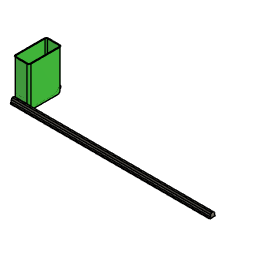
main v3 (Autodesk Fusion 360 archive; units mm, degrees)
design "main"
part number: Configuration 1
Autodesk Fusion 360 part; units mm, degrees
sketch "Sketch1" plane through (0, 0, 0) normal (0, 0, 1) x (1, 0, 0)
  line L0 (0, 0) -> (24, 0)
  line L1 (24, 0) -> (24, 50)
  line L2 (24, 50) -> (0, 50)
  line L3 (0, 50) -> (0, 0)
  line L4 (0.25, 49.75) -> (23.75, 49.75)
  line L5 (23.75, 49.75) -> (23.75, 0.25)
  line L6 (23.75, 0.25) -> (0.25, 0.25)
  line L7 (0.25, 0.25) -> (0.25, 49.75)
  dimension "d5" = 24
  dimension "d6" = 50
  dimension "d8" = 0.25
  dimension "d9" = 0.25
  dimension "d10" = 0.25
  dimension "d11" = 0.25
  constraint horizontal L0
  constraint vertical L1
  constraint horizontal L2
  constraint vertical L3
  constraint coincident L0.start L3.end
  constraint horizontal L4
  constraint vertical L5
  constraint horizontal L6
  constraint vertical L7
  measures "d5" distance of L0.start L0.end
  measures "d6" distance of L0.start L2.end
  measures "d8" distance of L1 L5
  measures "d9" distance of L3 L7
  measures "d10" distance of L0 L6
  measures "d11" distance of L2 L4
extrude "Extrude1" add sketch "Sketch1" along normal blind 60 contours L4 L5 L6 L7 makes body 1
ref_plane "WorkPlane1" through (0, 25, 0) normal (0, 1, 0) x (0, 0, 1)
sketch "Sketch2" plane through (0, 0, 0) normal (1, 0, 0) x (0, 1, 0)
  line L0 (0, 0) -> (50, 0) construction
  line L1 (0, 0) -> (0, 5)
  line L2 (0, 5) -> (3, 5)
  line L3 (3, 5) -> (3, 2)
  line L4 (3, 2) -> (5, 0)
  line L5 (0, 0) -> (5, 0)
  line L6 (5.3536, 0) -> (3.25, 2.1036)
  line L7 (3.25, 2.1036) -> (3.25, 5.1036)
  line L8 (3.25, 5.1036) -> (0, 8.3536)
  line L9 (0, 8.3536) -> (0, 0)
  line L10 (5.3536, 0) -> (0, 0)
  line L11 (3, 5) -> (0, 8)
  line L12 (3, 5) -> (5.995, 5) construction
  line L13 (1.2, 6.8) -> (0, 6.8)
  line L14 (4.2, 0.8) -> (4.2, 0)
  dimension "d16" = 50
  dimension "d18" = 5
  dimension "d19" = 3
  dimension "d20" = 3
  dimension "d21" = 135
  dimension "d27" = 135
  dimension "d29" = 0.25
  dimension "d30" = 0.25
  dimension "d41" = 135
  dimension "d42" = 0.25
  dimension "d56" = 1.2
  dimension "d63" = 0.8
  constraint coincident L0.start L1.start
  constraint perpendicular L0 L1
  constraint perpendicular L1 L2
  constraint coincident L0 L4.end
  constraint coincident L0 L6.start
  constraint parallel L4 L6
  constraint vertical L0.start L8.end
  constraint horizontal L12
  constraint coincident L9 L11.end
  constraint coincident L11 L13.start
  constraint coincident L9 L13.end
  constraint perpendicular L9 L13
  constraint coincident L4 L14.start
  constraint coincident L5 L14.end
  constraint vertical L14
  measures "d16" distance of L0.start L0.end
  measures "d18" distance of L0.start L1.end
  measures "d19" distance of L1.end L2.end
  measures "d20" distance of L2.end L3.end
  measures "d21" angle of L3 L4
  measures "d27" angle of L7 L8
  measures "d29" distance of L4 L6
  measures "d30" distance of L3 L7
  measures "d41" angle of L11 L12
  measures "d42" distance of L8 L11
  measures "d56" distance of L13.start L13.end
  measures "d63" distance of L4.end L14
extrude "Extrude2" cut sketch "Sketch2" along normal through all and the other way through all bodies 1
extrude "Extrude3" add sketch "Sketch2" along normal blind 300 separate body contours L1 L2 L3 L4 L5 L9 L10 L14 | L2 L9 L11 L13 makes body 2
mirror "Mirror1" about plane through (0, 25, 0) normal (0, 1, 0) of "Extrude2", "Extrude3" makes body 3
sketch "Sketch3" plane through (0, 0, 0) normal (1, 0, 0) x (0, 1, 0)
  line L0 (0, 0) -> (50, 0) construction
  line L1 (50, 0) -> (50, 60) construction
  line L2 (50, 60) -> (0, 60)
  line L3 (0, 60) -> (0, 0) construction
  line L4 (48.55, 60) -> (48.55, 12.8)
  arc A0 (36.55, 0.8) -> (48.55, 12.8) centre (36.55, 12.8) ccw
  line L5 (36.55, 0.8) -> (13.45, 0.8)
  arc A1 (1.45, 12.8) -> (13.45, 0.8) centre (13.45, 12.8) ccw
  line L6 (1.45, 12.8) -> (1.45, 60)
  line L7 (0, 0) -> (50, 0)
  point P0 (3.25, 5.1036)
  dimension "d34" = 50
  dimension "d35" = 60
  dimension "d36" = 1.45
  dimension "d38" = 1.45
  dimension "d39" = 0.8
  dimension "d40" = 12
  constraint horizontal L0
  constraint vertical L1
  constraint horizontal L2
  constraint vertical L3
  constraint coincident L0.start L3.end
  constraint coincident L2 L4.start
  constraint perpendicular L2 L4
  constraint tangent L4 A0
  constraint perpendicular L4 L5
  constraint tangent L5 A1
  constraint coincident L2 L6.end
  constraint perpendicular L2 L6
  constraint tangent A0 L5
  constraint tangent A1 L6
  constraint equal A0 A1
  measures "d34" distance of L0.start L0.end
  measures "d35" distance of L0.start L2.end
  measures "d36" distance of L1 L4
  measures "d38" distance of L3 L6
  measures "d39" distance of L5 L7
  measures "d40" radius of A1
extrude "Extrude4" cut sketch "Sketch3" along normal blind 21.1 from surface at 1.45 bodies 1
fillet "Fillet1" radius 1.8 10 edges at (1.45, 48.55, 36.4) (1.45, 45.0353, 4.3147) (1.45, 25, 0.8) (1.45, 4.9647, 4.3147) (1.45, 1.45, 36.4) (22.55, 1.45, 36.4) (22.55, 4.9647, 4.3147) (22.55, 25, 0.8) (22.55, 45.0353, 4.3147) (22.55, 48.55, 36.4) on bodies 1
fillet "Fillet1" radius 3 4 edges at (23.75, 0.25, 34.0518) (0.25, 0.25, 34.0518) (23.75, 49.75, 34.0518) (0.25, 49.75, 34.0518) on bodies 1
pattern_linear "R-Pattern4" count 2 spacing 50 along (0, -1, 0) of bodies 3 makes body 4
combine "Combine4" operation add target body 4 tool bodies 2
sketch "Sketch6" plane through (0, 0, 0) normal (0, 0, 1) x (1, 0, 0)
  circle A0 centre (50, 0) radius 1.3
  line L0 (0.25, -50) -> (-0.25, -50)
  line L1 (-0.25, -50) -> (-0.25, 50)
  line L2 (-0.25, 50) -> (0.25, 50)
  line L3 (0.25, 50) -> (0.25, -50)
  line L4 (0.25, -50) -> (-0.25, 50) construction
  line L5 (-0.25, -50) -> (0.25, 50) construction
  dimension "d91" = 2.6
  dimension "d92" = 50
  dimension "d93" = 0.5
  dimension "d94" = 100
  constraint horizontal origin A0.centre
  constraint horizontal L0
  constraint perpendicular L0 L1
  constraint parallel L0 L2
  constraint parallel L1 L3
  constraint coincident L4 origin
  constraint coincident L5 origin
  measures "d91" diameter of A0
  measures "d92" horizontal distance of origin A0.centre
  measures "d93" distance of L1.end L2.end
  measures "d94" distance of L0.end L1.end
extrude "Extrude9" cut sketch "Sketch6" along normal through all contours L0 L1 L2 L3 bodies 3 4
pattern_linear "R-Pattern5" count 2 spacing 300 along (1, 0, 0) of "Extrude9"
extrude "Extrude10" cut sketch "Sketch6" along normal blind 5 contours A0 bodies 4
pattern_linear "R-Pattern6" count 3 spacing 100 along (1, 0, 0) of "Extrude10"
sketch "Sketch7" plane through (0, 0, 0) normal (0, 0, 1) x (1, 0, 0)
  line L0 (0, 0) -> (300, 0)
  line L1 (300, 0) -> (300, 320)
  line L2 (300, 320) -> (0, 320)
  line L3 (0, 320) -> (0, 0)
  circle A0 centre (50, 10) radius 1.5
  circle A1 centre (50, 10) radius 3
  dimension "d109" = 300
  dimension "d110" = 320
  dimension "d114" = 3
  dimension "d115" = 50
  dimension "d116" = 10
  dimension "d123" = 6
  constraint horizontal L0
  constraint vertical L1
  constraint horizontal L2
  constraint vertical L3
  constraint coincident L0.start L3.end
  constraint concentric A0 A1
  measures "d109" distance of L0.start L0.end
  measures "d110" distance of L0.start L2.end
  measures "d114" diameter of A0
  measures "d115" horizontal distance of L0.start A0.centre
  measures "d116" vertical distance of L0.start A0.centre
  measures "d123" diameter of A1
extrude "Extrude11" add sketch "Sketch7" against normal blind 1 separate body contours L0 L1 L2 L3 | A0 | A1 makes body 5
extrude "Extrude13" add sketch "Sketch7" along normal blind 4 contours A1 bodies 5
chamfer "Chamfer1" distance 4 angle 45 1 edges at (47.203, 11.0848, 0) on bodies 5
extrude "Extrude12" cut sketch "Sketch7" against normal blind 57.976 contours A0 bodies 5
pattern_linear "R-Pattern7" count 3 spacing 100 along (1, 0, 0) count 7 spacing 50 along (0, 1, 0) of "Extrude13", "Chamfer1", "Extrude12"
copy_body "Body->Comp1" bodies 1 removing the originals makes body 6 in component "bin"
copy_body "Body->Comp2" bodies 3 removing the originals makes body 7 in component "track"
ref_plane "WorkPlane1" through (0, 50, 0) normal (0, 1, 0) x (0, 0, 1) in component "track"
mirror "Mirror1'" about plane through (0, 50, 0) normal (0, 1, 0) of bodies 7 merged in component "track"
pattern_linear "R-Pattern1" count 5 spacing 50 along (0, -1, 0) of bodies 7 makes body 8 at (100.0833, 1.4, 0) makes body 9 at (100.0833, -48.6, 0) makes body 10 at (100.0833, -98.6, 0) makes body 11 at (100.0833, -148.6, 0) in component "track"
sketch "Sketch1 (2)" plane through (0, 0, 0) normal (0, 0, 1) x (1, 0, 0) in component "track"
  line L0 (0.25, 54.2) -> (299.75, 54.2)
  line L1 (299.75, 54.2) -> (299.75, -154.2)
  line L2 (299.75, -154.2) -> (0.25, -154.2)
  line L3 (0.25, -154.2) -> (0.25, 54.2)
  line L4 (0.25, 51.5) -> (6.25, 51.5)
  line L5 (6.25, 51.5) -> (6.25, 48.5)
  line L6 (6.25, 48.5) -> (0.25, 48.5)
  line L7 (0.25, 48.5) -> (0.25, 51.5)
  line L8 (0.25, 54.2) -> (0.25, 45.8) construction
  line L9 (0.25, 50) -> (3.4309, 50) construction
  line L10 (150, -154.2) -> (150, 54.2) construction
  line L11 (50, -154.2) -> (50, 54.2) construction
  line L12 (250, -154.2) -> (250, 54.2) construction
  line L13 (50, 50) -> (150, 50) construction
  line L14 (50, -150) -> (250, -150) construction
  circle A0 centre (50, -150) radius 1.3
  circle A1 centre (250, -150) radius 1.3
  line L15 (150, 50) -> (250, 50) construction
  circle A2 centre (250, 50) radius 1.3
  circle A3 centre (50, 50) radius 1.3
  point P0 (0.25, 54.2)
  point P1 (0.25, 45.8)
  dimension "d136" = 54.2
  dimension "d137" = 208.4
  dimension "d138" = 299.5
  dimension "d144" = 6
  dimension "d145" = 3
  dimension "d155" = 100
  dimension "d156" = 100
  dimension "d157" = 50
  dimension "d158" = 200
  dimension "d159" = 2.6
  constraint horizontal L0
  constraint vertical L1
  constraint horizontal L2
  constraint vertical L3
  constraint coincident P0 L0.start
  constraint horizontal L4
  constraint vertical L5
  constraint horizontal L6
  constraint vertical L7
  constraint coincident L3 L4.start
  constraint coincident P1 L8.end
  constraint midpoint L8 L9.start
  constraint perpendicular L7 L9
  constraint symmetric L4 L6 L9
  constraint midpoint L2 L10.start
  constraint midpoint L0 L10.end
  constraint coincident L2 L11.start
  constraint coincident L0 L11.end
  constraint perpendicular L0 L11
  constraint coincident L2 L12.start
  constraint coincident L0 L12.end
  constraint perpendicular L0 L12
  constraint coincident L11 L13.start
  constraint coincident L10 L13.end
  constraint perpendicular L10 L13
  constraint coincident L11 L14.start
  constraint coincident L12 L14.end
  constraint perpendicular L12 L14
  constraint coincident L14.start A0.centre
  constraint coincident L14.end A1.centre
  constraint coincident L12 L15.end
  constraint perpendicular L12 L15
  constraint coincident L15.end A2.centre
  constraint coincident L13.start A3.centre
  constraint equal A0 A1
  constraint equal A1 A2
  constraint equal A2 A3
  measures "d136" vertical distance of origin L0.start
  measures "d137" distance of P0 L2.end
  measures "d138" distance of P0 L0.end
  measures "d144" distance of L4.start L4.end
  measures "d145" distance of L4.start L6.end
  measures "d155" distance of L10 L11
  measures "d156" distance of L10 L12
  measures "d157" distance of origin L13
  measures "d158" distance of L13 L14
  measures "d159" diameter of A0
extrude "Extrude1'" add sketch "Sketch1 (2)" against normal blind 0.4 contours L0 L1 L2 L3 L4 L5 L6 | L3 L4 L5 L6 L7 | A0 | A1 | A2 | A3 bodies 7 8 9 10 11 in component "track"
extrude "Extrude2'" cut sketch "Sketch1 (2)" along normal blind 4 from surface at -0.4 contours L3 L4 L5 L6 L7 bodies 7 in component "track"
ref_plane "WorkPlane2" through (150, -50, 3.2) normal (-1, 0, 0) x (0, -1, 0) in component "track"
mirror "Mirror2" about plane through (150, -50, 3.2) normal (-1, 0, 0) of "Extrude2'" in component "track"
pattern_linear "R-Pattern2" count 5 spacing 50 along (0, -1, 0) of "Extrude2'", "Mirror2" in component "track"
extrude "Extrude3'" cut sketch "Sketch1 (2)" against normal through all and the other way through all contours A0 | A1 | A2 | A3 bodies 7 in component "track"
component "bin" placed x (1, 0, 0) y (0, 1, 0) z (0, 0, 1) at (0, 0, 0)
component "track" placed x (1, 0, 0) y (0, 1, 0) z (0, 0, 1) at (0, 0, 0)
hidden bodies 5
equation "unitWidth = 12 mm"
equation "height = 50 mm"
equation "width = 2" comment "2,3,4,..."
equation "d5 = unitWidth * width"
equation "d6 = height"
equation "binBinTolerance = 0.5 mm"
equation "d8 = binBinTolerance / 2"
equation "d9 = binBinTolerance / 2"
equation "d10 = binBinTolerance / 2"
equation "d11 = binBinTolerance / 2"
equation "depth = 60 mm"
equation "roundedRadius = 3 mm"
equation "d14 = depth"
equation "d16 = height"
equation "d24 = height / 2"
equation "binTrackTolerance = 0.25 mm"
equation "d29 = binTrackTolerance"
equation "d30 = binTrackTolerance"
equation "d32 = trackWidth"
equation "d34 = height"
equation "d35 = depth"
equation "d36 = binBinTolerance / 2 + wallThickness"
equation "wallThickness = 1.2 mm"
equation "d38 = d36"
equation "d42 = binTrackTolerance"
equation "d43 = binBinTolerance / 2 + wallThickness"
equation "d44 = unitWidth * width - binBinTolerance - wallThickness * 2"
equation "d47 = roundedRadius - wallThickness"
equation "d49 = roundedRadius"
equation "copies = 2"
equation "trackWidth = 300 mm"
equation "trackWidthTolerance = 0.5 mm"
equation "trackScrewSpacing = 100 mm"
equation "trackScrewDiameter = 2.6 mm"
equation "d89 = -height"
equation "d91 = trackScrewDiameter"
equation "d92 = trackScrewSpacing / 2"
equation "d93 = trackWidthTolerance"
equation "trackScrewDepth = 5 mm"
equation "d99 = trackWidth"
equation "d101 = trackScrewDepth"
equation "d103 = trackWidth / trackScrewSpacing"
equation "d105 = trackScrewSpacing"
equation "drillGuideX = 300 mm"
equation "drillGuideY = 320 mm"
equation "d109 = drillGuideX"
equation "d110 = drillGuideY"
equation "drillGuideScrewDiameter = 3 mm"
equation "d114 = drillGuideScrewDiameter"
equation "d115 = trackScrewSpacing / 2"
equation "d119 = ceil(drillGuideX / trackScrewSpacing)"
equation "d120 = ceil(drillGuideY / height)"
equation "d121 = trackScrewSpacing"
equation "d122 = height"
equation "trackTileWidth = 300 mm"
equation "trackTileCopies = 5"
equation "d129 = height"
equation "d132 = trackTileCopies"
equation "d134 = -height"
equation "d137 = height * trackTileCopies - height + ( d136 - height ) * 2"
equation "d138 = trackTileWidth - trackWidthTolerance"
equation "d151 = trackTileCopies"
equation "d153 = height"
equation "d155 = trackScrewSpacing"
equation "d156 = d155"
equation "d157 = height"
equation "d158 = height * trackTileCopies - height"
equation "d159 = trackScrewDiameter"
named bodies: "bin", "track single", "drill guide"
